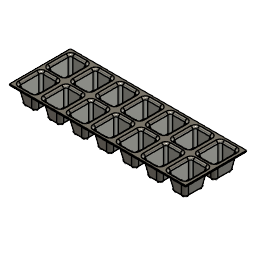
Day 5 Ice Cube Tray (Autodesk Fusion 360 design; units mm, degrees)
part number: 2026-07-05-03-32-47-395
Autodesk Fusion 360 part; units mm, degrees
sketch "Sketch1" plane through (0, 0, 0) normal (0, 1, 0) x (1, 0, 0)
  line L0 (150, 52) -> (-150, 52)
  line L1 (-150, 52) -> (-150, -52)
  line L2 (-150, -52) -> (150, -52)
  line L3 (150, -52) -> (150, 52)
  line L4 (150, 52) -> (-150, -52) construction
  line L5 (-150, 52) -> (150, -52) construction
  dimension "d1" = 300
  dimension "d2" = 104
  constraint horizontal L0
  constraint perpendicular L0 L1
  constraint parallel L0 L2
  constraint parallel L1 L3
  constraint coincident L4 origin
  constraint coincident L5 origin
  measures "d1" distance of L1.end L2.end
  measures "d2" distance of L0.end L1.end
extrude "Extrude1" add sketch "Sketch1" along normal blind 50
sketch "Sketch2" plane through (0, 50, 0) normal (0, 1, 0) x (-1, 0, 0)
  line L0 (-150, 52) -> (-150, -52)
  line L1 (-150, -52) -> (150, -52)
  line L2 (150, -52) -> (150, 52)
  line L3 (150, 52) -> (-150, 52)
  line L4 (143, -45) -> (113, -45)
  line L5 (113, -45) -> (113, -5)
  line L6 (113, -5) -> (143, -5)
  line L7 (143, -5) -> (143, -45)
  dimension "d5" = 30
  dimension "d6" = 40
  dimension "d7" = 7
  dimension "d8" = 7
  constraint horizontal L4
  constraint vertical L5
  constraint horizontal L6
  constraint vertical L7
  measures "d5" distance of L4.start L4.end
  measures "d6" distance of L4.start L6.end
  measures "d7" distance of L1 L4
  measures "d8" distance of L2 L7
extrude "Extrude2" cut sketch "Sketch2" against normal blind 30 draft -10 contours L4 L5 L6 L7
fillet "Fillet1" radius 4 5 faces at (-124.7633, 20, -20.0966) (-141.2367, 40, -20.0966) (-124.7633, 40, -6.7633) (-114.7633, 40, -29.9034) (-131.2367, 40, -43.2367)
pattern_linear "R-Pattern1" count 7 spacing 42.5 along (1, 0, 0) count 2 spacing 50 along (0, 0, 1) of "Extrude2", "Fillet1"
shell "Shell1" thickness 2 removed faces 5 at (-50, 16.6667, 52) at (-150, 16.6667, -17.3333) at (50, 16.6667, -52) at (150, 16.6667, 17.3333) at (-50, 0, 17.3333)
sketch "Sketch3" plane through (0, 0, 0) normal (0, 0, 1) x (1, 0, 0)
  point P0 (-150, 50)
equation "d8 = d7"
